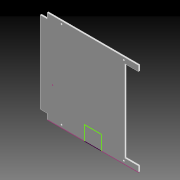
# Autodesk Inventor part: KB33-046-004-018 - Полка электроники
Saved by Autodesk Inventor 2020 (Build 240168000, 168)
## iProperties
Created: 2021-06-26
Part Number: KB33-046-004-018 - Полка электроники
Material: Типовые
Document SubType Name: Modeling
Designer: Петров Иван
Mass: 225.338 g
Surface Area: 1180.06 cm^2
Volume: 225.338 cm^3
Density: 1 g/cm^3
Appearance: По умолчанию
Author: Петров Иван
Autodesk Inventor part; units mm, degrees
ref_plane "YZ Plane" through (0, 0, 0) normal (1, 0, 0) x (0, 1, 0)
ref_plane "XZ Plane" through (0, 0, 0) normal (0, 1, 0) x (-1, 0, 0)
ref_plane "XY Plane" through (0, 0, 0) normal (0, 0, 1) x (1, 0, 0)
sketch "Эскиз1" plane through (0, 0, 0) normal (0, 0, 1) x (1, 0, 0)
  circle A0 centre (25, 157.5) radius 2
  circle A1 centre (196.5682, 157.5) radius 2
  line L0 (236.5682, 150) -> (236.5682, 165) projected
  line L1 (-34.0192, 150) -> (-15, 150)
  line L2 (-34.0192, 150) -> (-15, 150)
  line L3 (-34.0192, 37.5) -> (-34.0192, 150)
  line L4 (236.5682, 165) -> (-15, 165)
  line L5 (236.5682, 37.5) -> (236.5682, 165)
  line L6 (-34.0192, 37.5) -> (236.5682, 37.5)
  line L7 (-15, 165) -> (-15, 150)
  dimension "d5" = 127.5
  dimension "d6" = 7.5
  dimension "d7" = 7.5
  dimension "d9" = 15
  constraints: 14 end point, 2 centre point, 1 horizontal, 1 vertical
  measures "d5" distance between parallel lines of L6 L4
  measures "d6" distance from line of L4 A1.centre
  measures "d7" distance from line of L4 A0.centre
  measures "d9" distance of L4.end L1.end
extrude "Выдавливание1" add sketch "Эскиз1" along normal blind 4
sketch "Эскиз2" plane through (0, 0, 4) normal (0, 0, 1) x (1, 0, 0)
  line L0 (236.5682, 150) -> (199.2972, 150)
  line L1 (-15, 150) -> (-34.0192, 150) projected
  line L2 (-34.0192, 37.5) -> (236.5682, 37.5) projected
  line L3 (199.2972, 150) -> (236.5682, 150)
  line L4 (236.5682, 150) -> (236.5682, 37.5)
  line L5 (236.5682, 37.5) -> (199.2972, 37.5)
  line L6 (199.2972, 37.5) -> (199.2972, 150)
  point P0 (0, 0)
  point P1 (-24.5096, 150)
  point P2 (-15, -15)
  constraints: 10 end point, 2 horizontal, 2 parallel, 1 horizontal alignment, 1 midpoint, 1 perpendicular
extrude "Выдавливание2" cut sketch "Эскиз2" against normal blind 4
mirror "Зеркальное отражение2" about plane through (-34.0192, 37.5, 0) normal (0, -1, 0) of "Выдавливание1", "Выдавливание2"
sketch "Эскиз3" plane through (0, 0, 4) normal (0, 0, 1) x (1, 0, 0)
  line L0 (236.5682, -90) -> (-15, -90) projected
  line L1 (87.4676, -90) -> (133.662, -90)
  line L2 (133.662, -90) -> (133.662, -50.4003)
  line L3 (133.662, -50.4003) -> (87.4676, -50.4003)
  line L4 (87.4676, -50.4003) -> (87.4676, -90)
  point P0 (0, 0)
  constraints: 8 end point, 2 parallel, 1 horizontal, 1 perpendicular, 1 point on line
extrude "Выдавливание3" cut sketch "Эскиз3" against normal blind 10
ref_plane "РабПлоскость1" through (199.2972, 37.5, 4) normal (0, 1, 0) x (1, 0, 0)
mirror "Зеркальное отражение3" about plane through (199.2972, 37.5, 4) normal (0, 1, 0) of "Выдавливание3"
